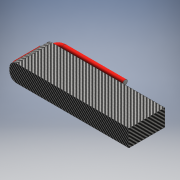
# Autodesk Inventor part: Battery_LI polymer_30C
Saved by Autodesk Inventor 2016 (Build 200138000, 138)
## iProperties
Created: 2019-09-19
Part Number: Battery_LI polymer_30C
Material: Generic
Document SubType Name: Modeling
Designer: jimmy
Density: 1 g/cm^3
Appearance: Default
Author: jimmy
Autodesk Inventor part; units mm, degrees
ref_plane "XZ Plane" through (0, 0, 0) normal (0, 1, 0) x (-1, 0, 0)
ref_plane "XY Plane" through (0, 0, 0) normal (0, 0, 1) x (1, 0, 0)
sketch "Sketch1" plane through (0, 0, 0) normal (0, 0, 1) x (1, 0, 0)
  line L0 (-70, -21) -> (70, -21)
  line L1 (70, -21) -> (70, 21)
  line L2 (70, 21) -> (-70, 21)
  line L3 (-70, 21) -> (-70, -21)
  line L4 (-70, -21) -> (70, 21) construction
  line L5 (70, -21) -> (-70, 21) construction
  point P0 (0, 0)
  dimension "d0" = 140
  dimension "d1" = 42
  constraints: 12 end point, 2 midpoint, 2 parallel, 1 horizontal, 1 perpendicular
  measures "d0" distance of L2.end L1.end
  measures "d1" distance of L1.end L0.end
extrude "Extrusion1" add sketch "Sketch1" along normal mid plane 20
sketch "Sketch2" plane through (-70, 21, 10) normal (0, 1, 0) x (1, 0, 0)
  line L0 (0, 20) -> (0, 0) projected
  line L1 (140, 0) -> (0, 0) projected
  line L2 (140, 20) -> (140, 0) projected
  line L3 (0, 20) -> (140, 20) projected
  line L4 (0, 20) -> (0, 0) construction
  line L5 (0, 10) -> (140, 10) construction
  circle A0 centre (7, 15.0139) radius 2.75
  circle A1 centre (7, 4.9861) radius 2.75
  line L6 (7, 4.9861) -> (7, 15.0139) construction
  point P0 (70, 10)
  point P1 (7, 10)
  dimension "d4" = 5.5
  dimension "d5" = 5.5
  dimension "d6" = 7
  constraints: 4 end point, 3 midpoint, 2 centre point, 1 point on line, 1 vertical
  measures "d4" diameter of A0
  measures "d5" diameter of A1
  measures "d6" distance between parallel lines of L0 L6
sketch "Sketch3" plane through (0, 0, 0) normal (0, 0, 1) x (1, 0, 0)
  arc A0 (-55.4861, 28.5139) -> (-63, 21) centre (-55.4861, 21) ccw
  line L0 (70, 21) -> (-70, 21) projected
  line L1 (-55.4861, 28.5139) -> (16.0285, 28.5139)
  point P0 (0, 0)
  constraints: 2 end point, 2 point on circle, 1 centre point, 1 horizontal, 1 line through centre, 1 tangent
sweep "Sweep1" add profiles "Sketch2" path "Sketch3" path curves A0 L1 contours A0 | A1
fillet "Fillet1" radius 8 2 edges at (-70, 0, -10) (-70, 0, 10)
ref_plane "Work Plane1" through (-62, 21, 10) normal (-1, 0, 0) x (0, -1, 0)
sketch "Sketch4" plane through (-62, 21, 10) normal (-1, 0, 0) x (0, -1, 0)
  line L0 (0, -20) -> (0, 0) projected
  line L1 (42, 0) -> (0, 0) projected
  line L2 (42, -20) -> (42, 0) projected
  line L3 (0, -20) -> (42, -20) projected
  line L4 (0, -20) -> (0, 0) construction
  line L5 (0, -10) -> (42, -10) construction
  circle A0 centre (40.4396, -12.25) radius 0.75
  circle A1 centre (40.4396, -10.75) radius 0.75
  circle A2 centre (40.4396, -7.75) radius 0.75
  circle A3 centre (40.4396, -9.25) radius 0.75
  point P0 (21, -10)
  dimension "d10" = 1.5
  dimension "d11" = 1.5
  dimension "d12" = 0.75
  dimension "d13" = 1.5
  constraints: 4 centre point, 2 end point, 2 midpoint, 2 symmetric about line, 2 other
  measures "d10" diameter of A0
  measures "d11" diameter of A1
  measures "d12" distance from line of L5 A1.centre
  measures "d13" distance of A1.centre A0.centre
sketch "Sketch5" plane through (0, 0, 0) normal (0, 0, 1) x (1, 0, 0)
  line L0 (-72.8899, 17.6929) -> (-72.8899, -11.4397)
  line L1 (-101.4679, 0) -> (98.578, 0) construction
  line L2 (0, -31.4528) -> (0, 41.7167) construction
  arc A0 (-72.8899, -11.4397) -> (-62, -19.4396) centre (-64.5065, -11.4397) ccw
  point P0 (0, 0)
  constraints: 2 end point, 2 point on circle, 1 centre point, 1 parallel, 1 tangent, 1 vertical
sweep "Sweep2" add profiles "Sketch4" path "Sketch5" path curves A0 L0 contours A0 | A2 | A3 | A1
body "Solid1"
